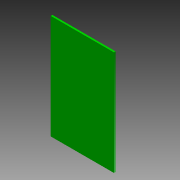
# Autodesk Inventor part: TableMount-Holder
Saved by Autodesk Inventor 2012 (Build 160160000, 160)
## iProperties
Created: 2013-07-16
Part Number: TableMount-Holder
Material: ABS Plastic
Document SubType Name: Modeling
Designer: joe_000
Density: 1.06 g/cm^3
Mass: 86.3684 g
Surface Area: 514.568 cm^2
Volume: 81.4797 cm^3
Author: joe_000
Autodesk Inventor part; units mm, degrees
ref_plane "YZ Plane" through (0, 0, 0) normal (1, 0, 0) x (0, 1, 0)
ref_plane "XZ Plane" through (0, 0, 0) normal (0, 1, 0) x (-1, 0, 0)
ref_plane "XY Plane" through (0, 0, 0) normal (0, 0, 1) x (1, 0, 0)
sketch "Sketch1" plane through (0, 0, 0) normal (0, 0, 1) x (1, 0, 0)
  line L0 (0, 0) -> (120, 0)
  line L1 (120, 0) -> (120, 198.5)
  line L2 (120, 198.5) -> (0, 198.5)
  line L3 (0, 198.5) -> (0, 0)
  dimension "d0" = 120
  dimension "d1" = 198.5
  constraints: 8 end point, 2 parallel, 1 horizontal, 1 perpendicular
  measures "d0" distance of L1.end L2.end
  measures "d1" distance of L0.end L1.end
extrude "Extrusion1" add sketch "Sketch1" along normal blind 3.175
ref_plane "Work Plane1" through (60, 0, 0) normal (1, 0, 0) x (0, 0, -1)
sketch "Sketch2" plane through (60, 0, 0) normal (1, 0, 0) x (0, 0, -1)
  line L0 (0, 161.8288) -> (19.05, 157.6055)
  line L1 (0, 136.4288) -> (19.05, 140.6521)
  line L2 (0, 178.6416) -> (0, 113.5366)
  arc A0 (19.05, 140.6521) -> (19.05, 157.6055) centre (17.1708, 149.1288) ccw
  circle A1 centre (17.1708, 149.1288) radius 3.175
  line L3 (0, 0) -> (0, 198.5) projected
  dimension "d4" = 25.4
  dimension "d7" = 19.05
  dimension "d8" = 102.5
  dimension "d9" = 102.5
  dimension "d10" = 6.35
  constraints: 6 end point, 3 point on line, 2 centre point, 2 point on circle, 1 coincident, 1 tangent, 1 vertical, 1 vertical alignment
  measures "d4" distance of L1.start L0.start
  measures "d7" horizontal distance of L1.start L1.end
  measures "d8" angle of L3 L0
  measures "d9" angle of L3 L1
  measures "d10" diameter of A1
extrude "Extrusion2" add sketch "Sketch2" along normal mid plane 12.2
fillet "Fillet1" radius 3.175 2 edges at (60, 136.4288, 0) (60, 161.8288, 0)
ref_plane "Work Plane2" through (93.02, 0, 0) normal (1, 0, 0) x (0, 0, -1)
sketch "Sketch3" plane through (93.02, 0, 0) normal (1, 0, 0) x (0, 0, -1)
  line L0 (0, 33.6062) -> (6.35, 32.1985)
  line L1 (0, 23.3513) -> (6.35, 24.7591)
  line L2 (0, 0) -> (0, 198.5) projected
  arc A0 (6.35, 24.7591) -> (6.35, 32.1985) centre (5.5254, 28.4788) ccw
  circle A1 centre (5.5254, 28.4788) radius 0.635
  circle A2 centre (17.1708, 149.1288) radius 3.175 projected
  line L3 (0, 33.6062) -> (0, 23.3513)
  dimension "d14" = 6.35
  dimension "d15" = 102.5
  dimension "d16" = 102.5
  dimension "d17" = 1.27
  dimension "d18" = 3.175
  dimension "d19" = 120.65
  constraints: 6 end point, 2 centre point, 2 point on circle, 2 vertical alignment, 1 coincident, 1 collinear, 1 point on line, 1 tangent
  measures "d14" horizontal distance of L0.start L0.end
  measures "d15" angle of L2 L0
  measures "d16" angle of L2 L1
  measures "d17" diameter of A1
  measures "d18" radial gap between concentric circles of A0 A1
  measures "d19" vertical distance of A2.centre A1.centre
extrude "Extrusion3" add sketch "Sketch3" along normal mid plane 3.175 contours L0 A0 L1 L2
fillet "Fillet2" radius 3.175 2 edges at (93.02, 33.6062, 0) (93.02, 23.3513, 0)
equation "\"d0\" = TabletWidth"
equation "\"d1\" = TabletHeight"
equation "\"d4\" = PivotWidth"
equation "\"d7\" = PivotHeight"
equation "\"d8\" = PivotAngle"
equation "\"d9\" = PivotAngle"
equation "\"d10\" = PivotScrewDiameter"
equation "\"d15\" = PivotAngle"
equation "\"d16\" = PivotAngle"
equation "\"TabletWidth\" = 120"
equation "\"TabletHeight\" = 198.5"
equation "\"PivotWidth\" = 25.4"
equation "\"PivotHeight\" = 19.05"
equation "\"PivotAngle\" = 102.5deg"
equation "\"PivotScrewDiameter\" = 6.35"
body "Solid1"
